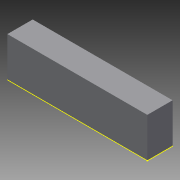
# Autodesk Inventor part: Součást1
Saved by Autodesk Inventor 2014 (Build 180170000, 170)
## iProperties
Created: 2015-09-26
Part Number: Součást1
Material: Všeobecné
Document SubType Name: Modeling
Designer: N
Density: 1 g/cm^3
Appearance: Výchozí
Author: N
Autodesk Inventor part; units mm, degrees
ref_plane "YZ Plane" through (0, 0, 0) normal (1, 0, 0) x (0, 1, 0)
ref_plane "XZ Plane" through (0, 0, 0) normal (0, 1, 0) x (-1, 0, 0)
ref_plane "XY Plane" through (0, 0, 0) normal (0, 0, 1) x (1, 0, 0)
sketch "Náčrt1" plane through (0, 0, 0) normal (0, 1, 0) x (-1, 0, 0)
  point P0 (0, 0)
sketch "Náčrt2" plane through (0, 0, 0) normal (0, 1, 0) x (-1, 0, 0)
  line L0 (0, 0) -> (177, 0)
  line L1 (177, 0) -> (177, 50)
  line L2 (177, 50) -> (0, 50)
  line L3 (0, 50) -> (0, 0)
  constraints: 8 end point, 2 perpendicular, 1 horizontal, 1 parallel
extrude "Vysunutí1" add sketch "Náčrt2" along normal blind 2
sketch "Náčrt3" plane through (0, 2, 0) normal (0, 1, 0) x (1, 0, 0)
  line L0 (0, 0) -> (-177, 0) projected
  line L1 (-177, 0) -> (-177, -50) projected
  line L2 (-177, -50) -> (0, -50) projected
  line L3 (0, -50) -> (0, 0) projected
  line L4 (-177, 0) -> (-177, -2)
  line L5 (-175, -2) -> (-2, -2)
  line L6 (-177, -50) -> (-177, -48)
  line L7 (-175, -48) -> (-2, -48)
  line L8 (-177, -50) -> (-175, -50)
  line L9 (-175, -48) -> (-175, -2)
  line L10 (0, 0) -> (-2, 0)
  line L11 (-2, -2) -> (-2, -48)
  dimension "d4" = 2
  dimension "d5" = 2
  dimension "d6" = 2
  dimension "d7" = 2
  constraints: 16 end point, 4 perpendicular, 4 point on line
  measures "d4" distance of L0.end L4.end
  measures "d5" distance of L1.end L6.end
  measures "d6" distance of L1.end L8.end
  measures "d7" distance of L0.start L10.end
extrude "Vysunutí2" add sketch "Náčrt3" along normal blind 30
sketch "Náčrt4" plane through (0, 0, 0) normal (0, 0, -1) x (-1, 0, 0)
  line L0 (0, 0) -> (177, 0) projected
  line L1 (177, 0) -> (177, 32) projected
  line L2 (0, 32) -> (177, 32) projected
  line L3 (0, 0) -> (0, 32) projected
sketch "Náčrt5" plane through (0, 0, 0) normal (0, 0, -1) x (-1, 0, 0)
  line L0 (0, 0) -> (177, 0) projected
  line L1 (177, 0) -> (177, 32) projected
  line L2 (0, 32) -> (177, 32) projected
  line L3 (0, 0) -> (0, 32) projected
  line L4 (2, 2) -> (175, 2)
  line L5 (175, 2) -> (175, 32)
  line L6 (175, 32) -> (2, 32)
  line L7 (2, 32) -> (2, 2)
  constraints: 8 end point, 2 parallel, 1 horizontal, 1 perpendicular
